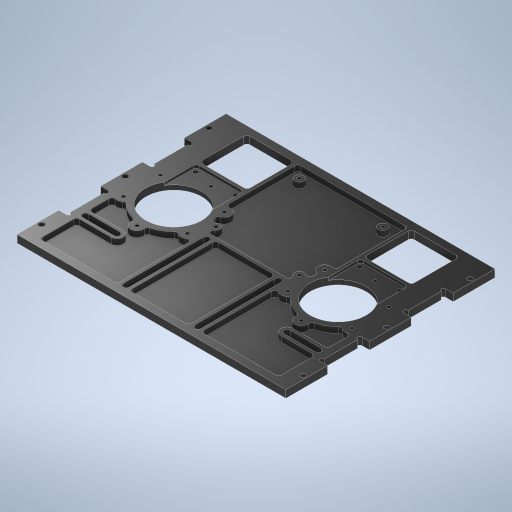
# Autodesk Inventor part: TorsoPelvisLowerFrame
Saved by Autodesk Inventor 2024.2 (Build 282272000, 272)
## iProperties
Created: 2024-01-05
Part Number: TorsoPelvisLowerFrame
Material: Aluminum 7075
Document SubType Name: Modeling
Designer: Masato Kubotera
Density: 2.81 g/cm^3
Appearance: Glossy - Black
Mass: 141.149 g
Surface Area: 518.013 cm^2
Volume: 50.2309 cm^3
Vendor: meviy
Author: Masato Kubotera
Autodesk Inventor part; units mm, degrees
ref_plane "YZ Plane" through (0, 0, 0) normal (1, 0, 0) x (0, 1, 0)
ref_plane "XZ Plane" through (0, 0, 0) normal (0, 1, 0) x (-1, 0, 0)
ref_plane "XY Plane" through (0, 0, 0) normal (0, 0, 1) x (1, 0, 0)
sketch "Sketch1" plane through (0, 0, 0) normal (0, 0, 1) x (1, 0, 0)
  line L0 (-70, -90) -> (70, -90)
  line L1 (70, -90) -> (70, 90)
  line L2 (70, 90) -> (-70, 90) construction
  line L3 (-70, 90) -> (-70, -90)
  line L4 (70, -90) -> (-70, 90) construction
  line L5 (-70, 0) -> (70, 0)
  line L6 (0, -90) -> (0, 90) construction
  circle A0 centre (0, 55) radius 18.75
  circle A1 centre (0, -55) radius 18.75
  line L7 (0, 55) -> (24.75, 55) construction
  circle A2 centre (0, 55) radius 29 construction
  line L8 (-31, 39) -> (12, 39) construction
  line L9 (12, 39) -> (12, 71) construction
  line L10 (12, 71) -> (-31, 71) construction
  line L11 (-31, 71) -> (-31, 39) construction
  line L12 (-31, 39) -> (12, 71) construction
  line L13 (12, 39) -> (-31, 71) construction
  line L14 (-28, 41.5) -> (-1, 41.5) construction
  line L15 (-1, 41.5) -> (-1, 68.5) construction
  line L16 (-1, 68.5) -> (-28, 68.5) construction
  line L17 (-28, 68.5) -> (-28, 41.5) construction
  line L18 (-28, 41.5) -> (-1, 68.5) construction
  line L19 (-1, 41.5) -> (-28, 68.5) construction
  line L20 (-9.6933, 38.95) -> (-31, 38.95)
  line L21 (-31, 38.95) -> (-31, 71.05)
  line L22 (-31, 71.05) -> (-9.6933, 71.05)
  line L23 (14, 90) -> (14, 85) construction
  line L24 (42, 85) -> (42, 90) construction
  line L25 (70, 87.5) -> (-70, 87.5) construction
  line L26 (13.95, 90) -> (13.95, 85)
  line L27 (42.05, 85) -> (42.05, 90)
  line L28 (28, 85) -> (28, 90) construction
  line L29 (13.95, 85) -> (42.05, 85)
  line L30 (-14, 90) -> (-14, 85) construction
  line L31 (-42, 85) -> (-42, 90) construction
  line L32 (-13.95, 90) -> (-13.95, 85)
  line L33 (-42.05, 85) -> (-42.05, 90)
  line L34 (-28, 85) -> (-28, 90) construction
  line L35 (-13.95, 85) -> (-42.05, 85)
  arc A3 (39.05, 85) -> (42.05, 85) centre (40.55, 85) ccw
  arc A4 (13.95, 85) -> (16.95, 85) centre (15.45, 85) ccw
  arc A5 (-42.05, 85) -> (-39.05, 85) centre (-40.55, 85) ccw
  arc A6 (-16.95, 85) -> (-13.95, 85) centre (-15.45, 85) ccw
  line L36 (25, 54) -> (47, 54) construction
  line L37 (47, 54) -> (47, -54) construction
  line L38 (47, -54) -> (25, -54) construction
  line L39 (25, -54) -> (25, 54) construction
  line L40 (25, 54) -> (47, -54) construction
  line L41 (47, 54) -> (25, -54) construction
  line L42 (-64, -35) -> (6, -35) construction
  line L43 (6, -35) -> (6, 35) construction
  line L44 (6, 35) -> (-64, 35) construction
  line L45 (-64, 35) -> (-64, -35) construction
  line L46 (-64, -35) -> (6, 35) construction
  line L47 (6, -35) -> (-64, 35) construction
  line L48 (-57, -28) -> (-1, -28) construction
  line L49 (-1, -28) -> (-1, 28) construction
  line L50 (-1, 28) -> (-57, 28) construction
  line L51 (-57, 28) -> (-57, -28) construction
  line L52 (-57, -28) -> (-1, 28) construction
  line L53 (-1, -28) -> (-57, 28) construction
  line L54 (-29, 35) -> (-29, -35) construction
  line L55 (5, 0) -> (5, 25)
  line L56 (-54.9493, -25.9493) -> (-3.0507, 25.9493) construction
  line L57 (7, 20) -> (7, -20)
  line L58 (65, -20) -> (65, 20)
  line L59 (65, 20) -> (7, 20)
  line L60 (65, 28) -> (65, 80)
  line L61 (65, 80) -> (14.6874, 80)
  line L62 (65, -20) -> (7, -20)
  line L63 (-65, 36.95) -> (-14.946, 36.95)
  line L64 (-33, 71.05) -> (-65, 71.05)
  line L65 (-65, 71.05) -> (-65, 38.95)
  line L66 (-65, 38.95) -> (-33, 38.95)
  line L67 (-33, 38.95) -> (-33, 71.05)
  line L68 (-33, 71.05) -> (-65, 38.95) construction
  line L69 (-65, 71.05) -> (-33, 38.95) construction
  arc A7 (22.2374, 51.5723) -> (22.2374, 58.4277) centre (24.75, 55) ccw
  arc A8 (14.0872, 72.5443) -> (14.6874, 80) centre (12.375, 76.4341) ccw
  arc A9 (14.5, 29.8853) -> (14.0872, 37.4557) centre (12.375, 33.5659) ccw
  arc A10 (-14.946, 36.95) -> (-8.1502, 34.028) centre (-12.375, 33.5659) ccw
  arc A11 (22.2374, 58.4277) -> (14.0872, 72.5443) centre (0, 55) ccw
  arc A12 (14.0872, 37.4557) -> (22.2374, 51.5723) centre (0, 55) ccw
  line L70 (-65, 0) -> (-65, 36.95)
  line L71 (-70, 90) -> (-42.05, 90)
  line L72 (-14, 90) -> (13.95, 90)
  line L73 (42.05, 90) -> (70, 90)
  arc A13 (62.95, 21.95) -> (62.95, 26.05) centre (62.95, 24) ccw
  line L74 (62.95, 24) -> (9.25, 24) construction
  arc A14 (9.25, 26.05) -> (9.25, 21.95) centre (9.25, 24) ccw
  line L75 (9.25, 21.95) -> (62.95, 21.95)
  line L76 (62.95, 26.05) -> (9.25, 26.05)
  line L77 (36.1, 56.85) -> (36.1, 77.95) construction
  arc A15 (34.05, 56.85) -> (38.15, 56.85) centre (36.1, 56.85) ccw
  arc A16 (38.15, 77.95) -> (34.05, 77.95) centre (36.1, 77.95) ccw
  line L78 (34.05, 56.85) -> (34.05, 77.95)
  line L79 (38.15, 77.95) -> (38.15, 56.85)
  circle A17 centre (12.375, 33.5659) radius 4.25 construction
  circle A18 centre (9.25, 24) radius 4 construction
  line L80 (12, 22.4123) -> (9.25, 20.8246) construction
  line L81 (9.25, 20.8246) -> (6.5, 22.4123) construction
  line L82 (6.5, 22.4123) -> (6.5, 25.5877) construction
  line L83 (6.5, 25.5877) -> (9.25, 27.1754) construction
  line L84 (9.25, 27.1754) -> (12, 25.5877) construction
  line L85 (12, 25.5877) -> (12, 22.4123) construction
  line L86 (10.583, 28) -> (65, 28)
  line L87 (12, -70) -> (60, -70) construction
  line L88 (60, -70) -> (60, 70) construction
  line L89 (60, 70) -> (12, 70) construction
  line L90 (12, 70) -> (12, -70) construction
  line L91 (12, -70) -> (60, 70) construction
  line L92 (60, -70) -> (12, 70) construction
  arc A19 (10.583, 28) -> (14.5, 29.8853) centre (0, 55) ccw
  arc A20 (32.1, 56.85) -> (40.1, 56.85) centre (36.1, 56.85) ccw
  line L93 (32.1, 56.85) -> (32.1, 80)
  line L94 (40.1, 56.85) -> (40.1, 80)
  line L95 (39.2754, 56.85) -> (37.6877, 54.1) construction
  line L96 (37.6877, 54.1) -> (34.5123, 54.1) construction
  line L97 (34.5123, 54.1) -> (32.9246, 56.85) construction
  line L98 (32.9246, 56.85) -> (34.5123, 59.6) construction
  line L99 (34.5123, 59.6) -> (37.6877, 59.6) construction
  line L100 (37.6877, 59.6) -> (39.2754, 56.85) construction
  line L101 (62.95, 27.1754) -> (65.7, 25.5877) construction
  line L102 (65.7, 25.5877) -> (65.7, 22.4123) construction
  line L103 (65.7, 22.4123) -> (62.95, 20.8246) construction
  line L104 (62.95, 20.8246) -> (60.2, 22.4123) construction
  line L105 (60.2, 22.4123) -> (60.2, 25.5877) construction
  line L106 (60.2, 25.5877) -> (62.95, 27.1754) construction
  arc A21 (40.1, 77.95) -> (32.1, 77.95) centre (36.1, 77.95) ccw construction
  circle A22 centre (-57, 28) radius 3
  arc A23 (-3.3939, 29.8081) -> (-4.5825, 32.9716) centre (-4.9898, 31.0135) ccw
  arc A24 (-8.1502, 34.028) -> (-4.5825, 32.9716) centre (0, 55) ccw
  arc A25 (5, 25) -> (1.4, 26.2) centre (3, 25) ccw
  arc A26 (-3.3939, 29.8081) -> (1.4, 26.2) centre (-1, 28) ccw
  point P0 (0, 0)
  point P1 (-12.375, 76.4341)
  point P2 (-24.75, 55)
  point P3 (12.375, 33.5659)
  point P4 (-9.5, 55)
  point P5 (-14.5, 55)
  point P6 (56, 87.5)
  point P7 (0, 87.5)
  point P8 (-56, 87.5)
  point P9 (-13.95, 90)
  point P10 (-42.05, 90)
  point P11 (-55.05, 85)
  point P12 (13.95, 85)
  point P13 (-13.95, 85)
  point P14 (36, 0)
  point P15 (-29, 0)
  point P16 (5, 0)
  point P17 (-39.05, 85)
  point P18 (-29, 0)
  point P19 (22.05, 32.9)
  point P20 (-49, 55)
  point P21 (16.95, 85)
  point P22 (-16.95, 85)
  dimension "d8" = 58
  dimension "d0" = 140
  dimension "d1" = 180
  dimension "d2" = 37.5
  dimension "d6" = 360
  dimension "d9" = 49.5
  dimension "d10" = 43
  dimension "d11" = 32
  dimension "d12" = 27
  dimension "d13" = 27
  dimension "d17" = 9.5
  dimension "d18" = 8.5
  dimension "d19" = 0.05
  dimension "d21" = 5
  dimension "d22" = 0.05
  dimension "d23" = 28
  dimension "d24" = 28
  dimension "d25" = 28
  dimension "d52" = 1.5
  dimension "d69" = 22
  dimension "d70" = 108
  dimension "d71" = 58
  dimension "d73" = 70
  dimension "d74" = 70
  dimension "d75" = 56
  dimension "d76" = 56
  dimension "d78" = 1
  dimension "d90" = 110
  dimension "d95" = 5
  dimension "d96" = 6
  dimension "d103" = 5
  dimension "d114" = 14
  dimension "d121" = 2
  dimension "d125" = 22.5
  dimension "d127" = 2
  dimension "d129" = 5
  dimension "d130" = 4.1
  dimension "d133" = 2
  dimension "d136" = 8
  dimension "d137" = 5.5
  dimension "d138" = 48
  dimension "d140" = 48
  dimension "d141" = 140
  dimension "d142" = 8
  dimension "d143" = 5.5
  dimension "d144" = 5.5
  dimension "d145" = 0.1
  dimension "d148" = 2
  dimension "d149" = 6
  constraints: 216 end point, 44 point on circle, 28 point on line, 26 midpoint, 25 centre point, 25 coincident, 24 symmetric about line, 20 parallel, 16 horizontal, 14 tangent, 14 vertical, 10 collinear, 9 perpendicular, 4 equal radius, 67 other
  measures "d0" distance of L2.end L1.end
  measures "d1" distance of L1.end L0.end
  measures "d2" diameter of A0
  measures "d9" distance of point (24.75, 55) point (-24.75, 55)
  measures "d10" distance of L10.end L9.end
  measures "d11" distance of L9.end L8.end
  measures "d12" distance of L16.end L15.end
  measures "d13" distance of L15.end L14.end
  measures "d17" distance from line of point (-9.5, 55) L6
  measures "d18" distance from line of L15 point (-9.5, 55)
  measures "d19" distance between parallel lines of L20 L8
  measures "d21" distance of L24.start L24.end
  measures "d22" distance between parallel lines of L27 L24
  measures "d23" distance between parallel lines of L23 L30
  measures "d24" distance between parallel lines of L1 L24
  measures "d25" distance between parallel lines of L24 L23
  measures "d52" radius of A3
  measures "d69" distance of L37.end L38.end
  measures "d70" distance of L36.end L37.end
  measures "d71" distance between parallel lines of L1 L9
  measures "d73" distance of L44.end L43.end
  measures "d74" distance of L43.end L42.end
  measures "d75" distance of L50.end L49.end
  measures "d76" distance of L49.end L48.end
  measures "d78" distance between parallel lines of L55 L43
  measures "d90" distance from line of L7 A1.centre
  measures "d95" distance between parallel lines of L1 L58
  measures "d96" distance between parallel lines of L45 L3
  measures "d103" distance between parallel lines of L61 L29
  measures "d114" distance from line of L1 point (56, 87.5)
  measures "d121" distance between parallel lines of L11 L67
  measures "d125" radius of A11
  measures "d127" distance between parallel lines of L63 L66
  measures "d129" distance between parallel lines of L65 L3
  measures "d130" diameter of A13
  measures "d133" distance between parallel lines of L57 L55
  measures "d136" diameter of A18
  measures "d137" distance between parallel lines of L85 L82
  measures "d138" diameter of L74 L5
  measures "d140" distance of L89.end L88.end
  measures "d141" distance of L88.end L87.end
  measures "d142" diameter of A20
  measures "d143" distance between parallel lines of L99 L96
  measures "d144" distance between parallel lines of L102 L105
  measures "d145" distance between parallel lines of L96 L36
  measures "d148" radius of A23
  measures "d149" diameter of A26
extrude "Extrusion1" add sketch "Sketch1" against normal blind 5 contours L3 L71 L33 A5 L35 A6 L32 L72 L26 A4 L29 A3 L27 L73 L1 L5 L58 L59 L57 L55 A25 A26 A23 A24 A10 L63 L70 | L70 L63 A10 A24 A23 A26 A25 L55 L5 | L5 L57 L59 L58 | A0 L20 L21 L22 | L86 A19 A9 A12 A7 A11 A8 L61 L93 A20 L94 L60 | L94 A20 L93 L61 | A22
extrude "Extrusion2" cut sketch "Sketch1" against normal blind 2 contours A0 L20 L21 L22
extrude "Extrusion3" cut sketch "Sketch1" against normal blind 4 contours L70 L63 A10 A24 A23 A26 A25 L55 L5 | L58 L62 L57 L5 | L5 L57 L59 L58 | L86 A19 A9 A12 A7 A11 A8 L61 L93 A20 L94 L60 | A16 L79 A15 L78
hole "Hole1" at (12.375, 33.5659, 0) at (-12.375, 33.5659, 0) at (24.75, 55, 0) at (12.375, 76.4341, 0) at (-12.375, 76.4341, 0) at (-24.75, 55, 0) at (-1, 28, 0) at (-57, 28, 0) direction (0, 0, -1) diameter 2.459 end through all thread size "M3x0.5" class "6H" standard "ANSI Metric M Profile"
hole "Hole2" at (56, 87.5, 0) at (0, 87.5, 0) at (-56, 87.5, 0) direction (0, 0, -1) diameter 3.5 end through all
hole "Hole3" at (-28, 41.5, 0) at (-28, 68.5, 0) direction (0, 0, -1) diameter 3.1 end through all
fillet "Fillet1" radius 2 21 edges at (-31, 38.95, -1) (-31, 71.05, -1) (65, 20, -2) (65, 80, -2) (14.6874, 80, -2) (7, 20, -2) (-65, 71.05, -2.5) (-33, 71.05, -2.5) (-33, 38.95, -2.5) (-65, 38.95, -2.5) (14.0872, 37.4557, -2) (14.0872, 72.5443, -2) (22.2374, 58.4277, -2) (22.2374, 51.5723, -2) (10.583, 28, -2) (32.1, 80, -2) (40.1, 80, -2) (65, 28, -2) (-8.1502, 34.028, -2) (-14.946, 36.95, -2) (-65, 36.95, -2)
mirror "Mirror1" about plane through (70, 0, 0) normal (0, -1, 0)
body "Solid1"
